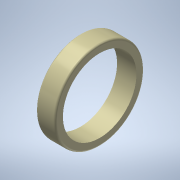
# Autodesk Inventor part: Rueda
Saved by Autodesk Inventor 2022.1 (Build 261234000, 234)
## iProperties
Created: 2021-09-22
Part Number: Rueda
Material: Genérico
Document SubType Name: Modeling
Designer: seb_0
Density: 1 g/cm^3
Appearance: Nilón 6
Author: seb_0
Autodesk Inventor part; units mm, degrees
ref_plane "YZ Plane" through (0, 0, 0) normal (1, 0, 0) x (0, 1, 0)
ref_plane "XZ Plane" through (0, 0, 0) normal (0, 1, 0) x (-1, 0, 0)
ref_plane "XY Plane" through (0, 0, 0) normal (0, 0, 1) x (1, 0, 0)
sketch "Boceto1" plane through (0, 0, 0) normal (1, 0, 0) x (0, 1, 0)
  circle A0 centre (0, 0) radius 115
  circle A1 centre (0, 0) radius 95
  dimension "d0" = 230
  dimension "d4" = 190
  constraints: 2 centre point, 2 coincident
  measures "d0" diameter of A0
  measures "d4" diameter of A1
extrude "Extrusión1" add sketch "Boceto1" along normal blind 50
fillet "Empalme1" radius 5 2 edges at (50, -115, 0) (0, -115, 0)
